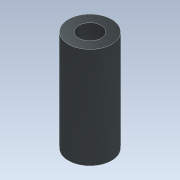
# Autodesk Inventor part: .875 in Grey Spacer
Saved by Autodesk Inventor 2021 (Build 250183000, 183)
## iProperties
Created: 2020-11-05
Part Number: .875 in Grey Spacer
Material: Nylon 6
Document SubType Name: Modeling
Designer: snake
Density: 1.12 g/cm^3
Appearance: Iron Gray
Author: snake
Autodesk Inventor part; units mm, degrees
ref_plane "YZ Plane" through (0, 0, 0) normal (1, 0, 0) x (0, 1, 0)
ref_plane "XZ Plane" through (0, 0, 0) normal (0, 1, 0) x (-1, 0, 0)
ref_plane "XY Plane" through (0, 0, 0) normal (0, 0, 1) x (1, 0, 0)
sketch "Sketch1" plane through (0, 0, 0) normal (0, 1, 0) x (-1, 0, 0)
  circle A0 centre (0, 0) radius 2.4638
  circle A1 centre (0, 0) radius 4.7625
  dimension "d0" = 4.9276
  dimension "d1" = 9.525
  constraints: 2 centre point, 2 coincident
  measures "d0" diameter of A0
  measures "d1" diameter of A1
extrude "Extrusion1" add sketch "Sketch1" along normal blind 22.225
body "Solid1"
